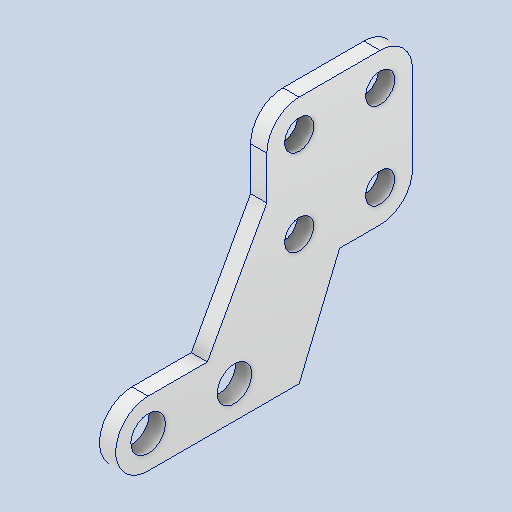
# Autodesk Inventor part: fork_inside
Saved by Autodesk Inventor 2024.1 (Build 281209000, 209)
## iProperties
Created: 2025-01-18
Part Number: fork_inside
Material: アルミニウム 6061
Document SubType Name: Sheet Metal
Designer: hibik
Density: 2.7 g/cm^3
Sheet Metal Rule: Default_mm
Appearance: アルミニウム - フラット
Author: hibik
Autodesk Inventor part; units mm, degrees
ref_plane "YZ Plane" through (0, 0, 0) normal (1, 0, 0) x (0, 1, 0)
ref_plane "XZ Plane" through (0, 0, 0) normal (0, 1, 0) x (-1, 0, 0)
ref_plane "XY Plane" through (0, 0, 0) normal (0, 0, 1) x (1, 0, 0)
sketch "スケッチ1" plane through (0, 0, 0) normal (1, 0, 0) x (0, 1, 0)
  line L0 (7, 0) -> (-7, 0)
  line L1 (-7, 0) -> (-7, -6.75)
  line L2 (-7, -6.75) -> (7, -6.75)
  line L3 (7, -6.75) -> (7, 0)
  circle A0 centre (4, -3.75) radius 3
  circle A1 centre (-4, -3.75) radius 3
  line L4 (7, -0.75) -> (-7, -0.75)
  line L5 (-6, -3.75) -> (-6, -14.75)
  line L6 (-6, -14.75) -> (6, -14.75)
  line L7 (6, -14.75) -> (6, -3.75)
  line L8 (-7, 0) -> (-7, 6.75)
  line L9 (-7, 6.75) -> (7, 6.75)
  line L10 (7, 6.75) -> (7, 0)
  circle A2 centre (4, 3.75) radius 3
  circle A3 centre (-4, 3.75) radius 3
  line L11 (7, 0.75) -> (-7, 0.75)
  circle A4 centre (4, -3.75) radius 1.35
  circle A5 centre (-4, -3.75) radius 1.35
  circle A6 centre (-4, 3.75) radius 1.35
  circle A7 centre (4, 3.75) radius 1.35
  circle A8 centre (3, -10.75) radius 1.6
  circle A9 centre (-3, -10.75) radius 1.6
  line L12 (0, -21.85) -> (0, 27.85)
  line L13 (-10, 20.75) -> (-16, 20.75)
  line L14 (-16, 20.75) -> (-16, 3.75)
  line L15 (-16, 3.75) -> (-10, 3.75)
  line L16 (-10, 3.75) -> (-10, 20.75)
  circle A10 centre (-13, 17.75) radius 1.6
  circle A11 centre (-13, 9.75) radius 1.6
  circle A12 centre (-13, 17.75) radius 3
  line L17 (-7, 0) -> (-16, 3.75)
  line L18 (0, 6.75) -> (-10, 12.25)
  point P0 (0, 0)
  point P1 (0, 0)
  point P2 (-4.1535, 3.75)
  point P3 (6, -5.9861)
  point P4 (7, -3.75)
  point P5 (7, 3.75)
  point P6 (-7, 3.75)
  point P7 (-7, -3.75)
  point P8 (-6, -5.9861)
  point P9 (4, 6.75)
  point P10 (-4, 6.75)
  point P11 (-16, 17.75)
  point P12 (-7, 6.75)
  point P13 (-1, 6.75)
  point P14 (-10, 17.75)
  point P15 (4, -6.75)
  point P16 (-4, -6.75)
  dimension "d0" = 14
  dimension "d1" = 6
  dimension "d2" = 6
  dimension "d3" = 0.75
  dimension "d4" = 8
  dimension "d5" = 2.7
  dimension "d7" = 3.2
  dimension "d8" = 3.2
  dimension "d9" = 4
  dimension "d10" = 6
  dimension "d11" = 3
  dimension "d12" = 6
  dimension "d13" = 3.2
  dimension "d14" = 3.2
  dimension "d15" = 3
  dimension "d16" = 8
  dimension "d17" = 3
  dimension "d18" = 3
  measures "d0" distance of L1.end L2.end
  measures "d1" diameter of A0
  measures "d2" diameter of A1
  measures "d3" distance between parallel lines of L0 L4
  measures "d4" distance between parallel lines of L6 L2
  measures "d5" diameter of A4
  measures "d7" diameter of A8
  measures "d8" diameter of A9
  measures "d9" distance from line of L2 A8.centre
  measures "d10" distance of A9.centre A8.centre
  measures "d11" distance from line of L7 A8.centre
  measures "d12" distance of L13.start L13.end
  measures "d13" diameter of A10
  measures "d14" diameter of A11
  measures "d15" distance from line of L9 A11.centre
  measures "d16" distance of A10.centre A11.centre
  measures "d17" distance from line of L13 A10.centre
  measures "d18" distance between parallel lines of L8 L16
extrude "プレート1" add sketch "スケッチ1" along normal blind 1.5 contours L3 L4 L12 L0 | L0 L12 L11 L10 | L12 L4 L1 L0 | L0 L8 L11 L12 | L3 A0 L4 | L11 A2 L10 | L17 L15 L16 L18 L9 L8 | L12 L2 A1 L4 | L4 A0 L2 L12 | L12 L9 A2 L11 | L11 A3 L9 L12 | A0 | A2 | L4 A1 L1 | L8 A3 L11 | L14 A12 L16 L15 | A1 | A3 | L8 L9 A3 | A12
equation "\"d11\" = 0.5 * d10"
equation "\"d17\" = 0.5 * d10"
equation "\"d6\" = Thickness"
equation "\"BendRadius\" = Thickness"
equation "\"BendReliefWidth\" = Thickness"
equation "\"BendReliefDepth\" = 0.5 * Thickness"
equation "\"CornerReliefSize\" = 4 * Thickness"
equation "\"MinimumRemnant\" = 2 * Thickness"
equation "\"TransitionRadius\" = BendRadius"
equation "\"JacobiRadiusSize\" = BendRadius"
equation "\"GapSize\" = Thickness"
equation "\"Thickness\" = 1.5"
